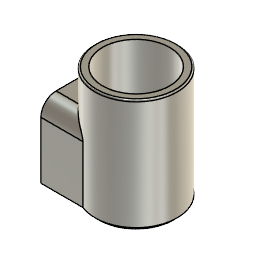
EchoWeather_AnemometerEnclosure (Autodesk Fusion 360 design; units mm, degrees)
Autodesk Fusion 360 part; units mm, degrees
sketch "Sketch1" plane through (0, 0, 0) normal (0, 0, 1) x (1, 0, 0)
  circle A0 centre (0, 0) radius 13.7922 construction
  circle A1 centre (0, 0) radius 13.6525
  circle A2 centre (0, 0) radius 11.1525
  dimension "d1" = 27.5844
  dimension "d2" = 27.305
  dimension "d3" = 2.5
  constraint coincident A0.centre A1.centre
  measures "d1" diameter of A0
  measures "d2" diameter of A1
  measures "d3" distance of A1 A2
extrude "Extrude1" add sketch "Sketch1" against normal blind 38.1 contours A1 | A2
sketch "Sketch2" plane through (0, 0, 0) normal (1, 0, 0) x (0, 1, 0)
  line L0 (0, 0) -> (0, -39.2845) construction
  circle A0 centre (0, -25.4) radius 9.525
  line L1 (0, 0) -> (-28.4764, 0) construction
  circle A1 centre (0, -25.4) radius 12.7 construction
  line L2 (-13.6525, -38.1) -> (13.6525, -38.1) construction
  line L3 (-12.7, -38.1) -> (12.7, -38.1)
  line L4 (12.7, -38.1) -> (12.7, -17.78)
  line L5 (7.62, -12.7) -> (-7.62, -12.7)
  line L6 (-12.7, -17.78) -> (-12.7, -38.1)
  line L7 (-12.7, -38.1) -> (12.7, -12.7) construction
  line L8 (12.7, -38.1) -> (-12.7, -12.7) construction
  arc A2 (12.7, -17.78) -> (7.62, -12.7) centre (7.62, -17.78) ccw
  arc A3 (-7.62, -12.7) -> (-12.7, -17.78) centre (-7.62, -17.78) ccw
  point P0 (0, -25.4)
  dimension "d6" = 19.05
  dimension "d8" = 25.4
  dimension "d9" = 5.08
  dimension "d10" = 5.08
  constraint coincident L0.start L1.start
  constraint vertical L0
  constraint coincident L0 P0
  constraint perpendicular L0 L1
  constraint concentric A0 A1
  constraint tangent A1 L2
  constraint horizontal L3
  constraint perpendicular L3 L4
  constraint parallel L3 L5
  constraint parallel L4 L6
  constraint coincident L7 P0
  constraint coincident L8 P0
  constraint coincident L2 L3.start
  constraint coincident P0 A0.centre
  constraint tangent A1 L6
  constraint coincident L7.end L5
  constraint coincident L7.end L4
  constraint tangent L5 A2
  constraint tangent L4 A2
  constraint coincident L8.end L5
  constraint coincident L8.end L6
  constraint tangent L5 A3
  constraint tangent L6 A3
  measures "d6" diameter of A0
  measures "d8" diameter of A1
  measures "d9" radius of A2
  measures "d10" radius of A3
extrude "Extrude2" add sketch "Sketch2" against normal blind 19.05
extrude "Extrude3" cut sketch "Sketch2" against normal blind 34.8234 contours A0
extrude "Extrude4" cut sketch "Sketch1" against normal up to surface (37.38 mm away) contours A2
fillet "Fillet1" radius 0.508 1 edges at (-12.7286, -4.937, 0)
chamfer "Chamfer1" distance 1.27 angle 45 1 faces at (1.1599, 0.6789, -38.1)
chamfer "Chamfer2" distance 0.762 angle 45 1 edges at (-19.05, -8.8804, -28.8444)
